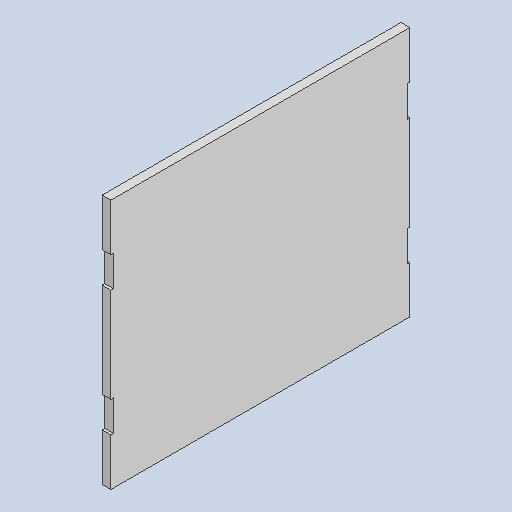
# Autodesk Inventor part: back_cowl
Saved by Autodesk Inventor 2025.2 (Build 292293000, 293)
## iProperties
Created: 2025-07-11
Part Number: back_cowl
Material: 일반
Document SubType Name: Modeling
Designer: jbhma
Density: 1 g/cm^3
Appearance: 기본값
Author: jbhma
Autodesk Inventor part; units mm, degrees
ref_plane "YZ Plane" through (0, 0, 0) normal (1, 0, 0) x (0, 1, 0)
ref_plane "XZ Plane" through (0, 0, 0) normal (0, 1, 0) x (-1, 0, 0)
ref_plane "XY Plane" through (0, 0, 0) normal (0, 0, 1) x (1, 0, 0)
sketch "스케치1" plane through (0, 0, 0) normal (1, 0, 0) x (0, 1, 0)
  line L0 (285, 170) -> (0, 170)
  line L1 (0, 170) -> (0, -170)
  line L2 (0, -170) -> (285, -170)
  line L3 (285, -170) -> (285, 170)
  point P0 (0, 0)
  point P1 (0, 0)
  dimension "d0" = 285
  dimension "d1" = 340
  constraints: 8 end point, 2 parallel, 1 coincident, 1 horizontal, 1 midpoint, 1 perpendicular
  measures "d0" distance between parallel lines of L3 L1
  measures "d1" distance of L0.end L1.end
extrude "돌출1" add sketch "스케치1" along normal blind 10
sketch "스케치2" plane through (10, 0, 0) normal (1, 0, 0) x (0, 0, -1)
  line L0 (-170, 0) -> (170, 0) construction
  line L1 (170, 0) -> (170, 285) construction
  line L2 (170, 285) -> (-170, 285) construction
  line L3 (-170, 285) -> (-170, 0) construction
  line L4 (-170, 142.5) -> (170, 142.5) construction
  line L5 (-170, 213.75) -> (170, 213.75) construction
  line L6 (-170, 71.25) -> (170, 71.25) construction
  line L7 (-170, 231.25) -> (-167, 231.25)
  line L8 (-167, 231.25) -> (-167, 196.25)
  line L9 (-167, 196.25) -> (-170, 196.25)
  line L10 (-170, 196.25) -> (-170, 231.25)
  line L11 (-170, 88.75) -> (-167, 88.75)
  line L12 (-167, 88.75) -> (-167, 53.75)
  line L13 (-167, 53.75) -> (-170, 53.75)
  line L14 (-170, 53.75) -> (-170, 88.75)
  line L15 (170, 88.75) -> (167, 88.75)
  line L16 (167, 88.75) -> (167, 53.75)
  line L17 (167, 53.75) -> (170, 53.75)
  line L18 (170, 53.75) -> (170, 88.75)
  line L19 (170, 231.25) -> (167, 231.25)
  line L20 (167, 231.25) -> (167, 196.25)
  line L21 (167, 196.25) -> (170, 196.25)
  line L22 (170, 196.25) -> (170, 231.25)
  point P0 (0, 0)
  point P1 (-167, 213.75)
  point P2 (-167, 71.25)
  point P3 (167, 71.25)
  point P4 (167, 213.75)
  dimension "d4" = 142.5
  dimension "d5" = 71.25
  dimension "d6" = 71.25
  dimension "d7" = 3
  dimension "d8" = 35
  dimension "d9" = 3
  dimension "d10" = 35
  dimension "d11" = 3
  dimension "d12" = 35
  dimension "d13" = 3
  dimension "d14" = 35
  constraints: 38 end point, 12 point on line, 8 parallel, 6 midpoint, 6 perpendicular, 4 horizontal
  measures "d4" distance between parallel lines of L2 L4
  measures "d5" distance between parallel lines of L2 L5
  measures "d6" distance between parallel lines of L0 L6
  measures "d7" distance of L8.end L9.end
  measures "d8" distance of L7.end L8.end
  measures "d9" distance of L12.end L13.end
  measures "d10" distance of L11.end L12.end
  measures "d11" distance of L17.end L16.end
  measures "d12" distance of L16.end L15.end
  measures "d13" distance of L21.end L20.end
  measures "d14" distance of L20.end L19.end
extrude "돌출2" cut sketch "스케치2" against normal blind 10
